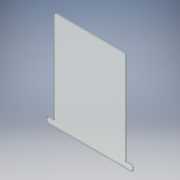
# Autodesk Inventor part: Tapa
Saved by Autodesk Inventor 2019 (Build 230136000, 136)
## iProperties
Created: 2020-04-07
Part Number: Tapa
Material: Generic
Document SubType Name: Modeling
Designer: Jurgen
Density: 1 g/cm^3
Appearance: Clear
Author: Jurgen
Autodesk Inventor part; units mm, degrees
ref_plane "YZ Plane" through (0, 0, 0) normal (1, 0, 0) x (0, 1, 0)
ref_plane "XZ Plane" through (0, 0, 0) normal (0, 1, 0) x (-1, 0, 0)
ref_plane "XY Plane" through (0, 0, 0) normal (0, 0, 1) x (1, 0, 0)
sketch "Sketch1" plane through (0, 0, 0) normal (0, 0, 1) x (1, 0, 0)
  line L0 (0, 0) -> (250, 0) construction
  line L1 (250, 0) -> (250, 345) construction
  line L2 (250, 345) -> (0, 345) construction
  line L3 (0, 345) -> (0, 0) construction
  line L4 (0, 0) -> (-25, 0) construction
  line L5 (-25, 0) -> (275, 0) construction
  line L6 (275, 0) -> (275, 20) construction
  line L7 (275, 20) -> (-25, 20) construction
  line L8 (-25, 20) -> (-25, 0) construction
  line L9 (275, 0) -> (-25, 0)
  line L10 (-25, 0) -> (-25, 20)
  line L11 (-25, 20) -> (0, 20)
  line L12 (0, 20) -> (0, 345)
  line L13 (0, 345) -> (250, 345)
  line L14 (250, 345) -> (250, 20)
  line L15 (250, 20) -> (275, 20)
  line L16 (275, 20) -> (275, 0)
  dimension "d0" = 250
  dimension "d2" = 25
  dimension "d3" = 300
  dimension "d7" = 325
  dimension "d8" = 20
  constraints: 34 end point, 5 perpendicular, 4 horizontal, 4 parallel, 4 point on line, 1 collinear, 1 vertical
  measures "d0" distance of L2.end L1.end
  measures "d2" distance of L0.start L4.end
  measures "d3" distance of L7.end L6.end
  measures "d7" distance between parallel lines of L2 L7
  measures "d8" distance of L5.end L6.end
extrude "Extrusion1" add sketch "Sketch1" along normal blind 3.5
fillet "Fillet1" radius 6 6 edges at (250, 345, 1.75) (0, 345, 1.75) (-25, 20, 1.75) (275, 20, 1.75) (275, 0, 1.75) (-25, 0, 1.75)
body "Solid1"
